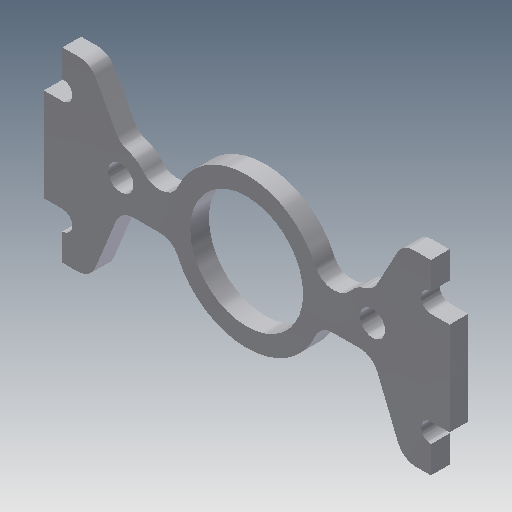
# Autodesk Inventor part: 足首_サブフレーム_1_2
Saved by Autodesk Inventor 2017.3 (Build 213256000, 256)
## iProperties
Created: 2016-04-30
Part Number: 足首_サブフレーム_1_2
Material: アルミニウム 2014-T4
Document SubType Name: Modeling
Designer: hiroaki
Density: 2.8 g/cm^3
Appearance: サテン
Mass: 1.79391 g
Surface Area: 10.4605 cm^2
Volume: 0.640682 cm^3
Author: hiroaki
Autodesk Inventor part; units mm, degrees
ref_plane "YZ Plane" through (0, 0, 0) normal (1, 0, 0) x (0, 1, 0)
ref_plane "XZ Plane" through (0, 0, 0) normal (0, 1, 0) x (-1, 0, 0)
ref_plane "XY Plane" through (0, 0, 0) normal (0, 0, 1) x (1, 0, 0)
sketch "スケッチ1" plane through (0, 0, 0) normal (0, 0, 1) x (1, 0, 0)
  circle A0 centre (0, 0) radius 10.5 construction
  circle A1 centre (-13.5, 1) radius 1.35
  line L0 (-13.5, 28) -> (13.5, 28) construction
  line L1 (13.5, 28) -> (13.5, 1) construction
  line L2 (13.5, 1) -> (-13.5, 1) construction
  line L3 (-13.5, 1) -> (-13.5, 28) construction
  circle A2 centre (-13.5, 28) radius 1.35
  circle A3 centre (13.5, 1) radius 1.35
  circle A4 centre (13.5, 28) radius 1.35
  line L4 (-19.75, 10) -> (-19.75, 7.1)
  line L5 (-19.75, 10) -> (19.75, 10)
  line L6 (19.75, 10) -> (19.75, 7.1)
  line L7 (-19.75, -7.1) -> (-19.75, -10)
  line L8 (-19.75, -10) -> (19.75, -10)
  line L9 (19.75, -7.1) -> (19.75, -10)
  line L10 (-19.75, 5) -> (-21.75, 5)
  line L11 (-21.75, 5) -> (-21.75, -5)
  line L12 (-21.75, -5) -> (-19.75, -5)
  arc A5 (-19.75, 5) -> (-19.75, 7.1) centre (-19.75, 6.05) ccw
  arc A6 (-19.75, -7.1) -> (-19.75, -5) centre (-19.75, -6.05) ccw
  line L13 (19.75, 5) -> (21.75, 5)
  line L14 (21.75, 5) -> (21.75, -5)
  line L15 (21.75, -5) -> (19.75, -5)
  arc A7 (19.75, 7.1) -> (19.75, 5) centre (19.75, 6.05) ccw
  line L16 (0, 28) -> (0, 0) construction
  arc A8 (19.75, -5) -> (19.75, -7.1) centre (19.75, -6.05) ccw
  line L17 (-21.75, 0) -> (21.75, 0) construction
  circle A9 centre (0, 0) radius 6.05
  point P0 (0, 10)
  dimension "d8" = 21
  dimension "d10" = 27
  dimension "d12" = 1
  dimension "d13" = 2.7
  dimension "d38" = 27
  dimension "d44" = 27
  dimension "d47" = 1.05
  dimension "d48" = 39.5
  dimension "d49" = 2
  dimension "d50" = 10
  dimension "d51" = 5
  dimension "d52" = 12.1
  constraints: 36 end point, 10 centre point, 9 perpendicular, 8 point on circle, 7 vertical alignment, 5 midpoint, 5 vertical, 4 horizontal, 4 tangent, 3 coincident, 3 equal radius, 2 parallel, 2 symmetric about line, 1 horizontal alignment, 8 other
  measures "d8" diameter of A0
  measures "d10" distance of L0.start L0.end
  measures "d12" distance from line of point (0, 0) L2
  measures "d13" diameter of A1
  measures "d38" distance of A1.centre A2.centre
  measures "d44" distance of A1.centre A3.centre
  measures "d47" radius of A5
  measures "d48" distance of L4.start L5.end
  measures "d49" distance between parallel lines of L11 L4
  measures "d50" distance between parallel lines of L12 L10
  measures "d51" distance between parallel lines of L5 L10
  measures "d52" diameter of A9
extrude "押し出し1" add sketch "スケッチ1" along normal blind 2 contours L5 L6 A7 L13 L14 L15 A8 L9 L8 L7 A6 L12 L11 L10 A5 L4
sketch "スケッチ2" plane through (0, 0, 2) normal (0, 0, 1) x (1, 0, 0)
  circle A0 centre (0, 0) radius 6.05 projected
  circle A1 centre (13.5, 1) radius 1.35 projected
  circle A2 centre (-13.5, 1) radius 1.35 projected
  line L0 (-19.75, -10) -> (19.75, -10) projected
  line L1 (21.75, -5) -> (21.75, 5) projected
  line L2 (19.75, 10) -> (-19.75, 10) projected
  line L3 (21.75, 0) -> (0, 0) construction
  line L4 (13.5, -2) -> (7.7976, -2)
  arc A3 (-7.7976, -2) -> (7.7976, -2) centre (0, 0) ccw
  line L5 (-13.5, -2) -> (-7.7976, -2)
  line L6 (0, 0) -> (0, -6.05) construction
  circle A4 centre (0, 0) radius 6.05 construction
  arc A5 (13.5, 4) -> (10.6716, 2) centre (13.5, 1) ccw
  line L7 (10.6716, 2) -> (7.7976, 2)
  arc A6 (7.7976, 2) -> (-7.7976, 2) centre (0, 0) ccw
  line L8 (-7.7976, 2) -> (-10.6716, 2)
  arc A7 (-10.6716, 2) -> (-13.5, 4) centre (-13.5, 1) ccw
  line L9 (-13.5, 4) -> (-18.2897, 12.8425)
  line L10 (-18.2897, 12.8425) -> (18.2897, 12.8425)
  line L11 (18.2897, 12.8425) -> (13.5, 4)
  line L12 (-13.5, -2) -> (-18.8131, -15.0783)
  line L13 (-18.8131, -15.0783) -> (18.8131, -15.0783)
  line L14 (18.8131, -15.0783) -> (13.5, -2)
  line L15 (-16.75, 10) -> (-19.75, 10) construction
  line L16 (16.75, 10) -> (19.75, 10) construction
  line L17 (-19.75, -10) -> (19.75, -10) construction
  line L18 (-19.75, -10) -> (-16.75, -10) construction
  line L19 (16.75, -10) -> (19.75, -10) construction
  dimension "d55" = 2
  dimension "d56" = 2
  dimension "d57" = 3
  dimension "d61" = 3
  dimension "d62" = 3
  constraints: 32 end point, 8 point on circle, 8 point on line, 6 horizontal, 5 symmetric about line, 4 centre point, 4 coincident, 4 vertical alignment, 3 collinear, 2 equal radius, 1 midpoint, 1 parallel, 1 vertical, 4 other
  measures "d56" distance between parallel lines of L3 L4
  measures "d57" radius of A5
  measures "d61" distance of L15.start L2.end
  measures "d62" distance of L0.start L18.end
extrude "押し出し2" cut sketch "スケッチ2" against normal blind 10 contours L12 L5 A3 L4 L14 L0 | L0 L14 L13 L12 | L11 A5 L7 A6 L8 A7 L9 L2
fillet "フィレット1" radius 2 14 edges at (7.7976, 2, 1) (7.7976, -2, 1) (-7.7976, -2, 1) (-7.7976, 2, 1) (13.5, -2, 1) (-13.5, -2, 1) (-13.5, 4, 1) (-10.6716, 2, 1) (10.6716, 2, 1) (13.5, 4, 1) (-16.75, 10, 1) (-16.75, -10, 1) (16.75, -10, 1) (16.75, 10, 1)
equation "\"d38\" = d10"
equation "\"d44\" = d10"
equation "\"d50\" = d11"
equation "\"d51\" = d12_1"
equation "\"d11\" = 10"
equation "\"d12_1\" = 5"
